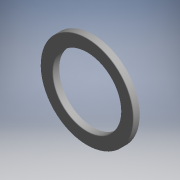
# Autodesk Inventor part: 51111 Housing raceway disc
Saved by Autodesk Inventor 2023 (Build 270158000, 158)
## iProperties
Part Number: 51111 Housing raceway disc
Material: 一般
Catalog Web Link: www.cadenas.de
Description: tb sdt hrd-
Vendor: NTN
Document SubType Name: Modeling
Designer: partserver
Manufacturer: NTN
Mass: 9.93491 g
Surface Area: 68.4869 cm^2
Volume: 9.93491 cm^3
Density: 1 g/cm^3
Appearance: PSOLRGB-192-192-192
Category: PARTsolutions
Company: NTN
PSOL_IDENT_0: {$CADENAS_DATA\23d-libs\ntn\ball_roller_bearings\thrust_b\tb_sdt_ir.prj},199 {VTYP=3D},{NB=51111 Hou
PSOL_IDENT_1: sing raceway disc},{LINA=51111 Housing raceway disc},{NN=tb sdt hrd},{DATE=21.12.2021 04:23:12},{GEO
PSOL_IDENT_2: MDATE=08.04.2020 13:27:59},{VERSION=},{LINEID=11140},{WBVAR=},{WBNUMERIC=}  {NB=51111 Housing racewa
PSOL_IDENT_3: y disc},{LINA=51111 Housing raceway disc},{KT=DUMMY},{IDNR=},{SD=55},{D=78},{T=16},{R=0.6},{ORDER=51
PSOL_IDENT_4: 111},{CA=35},{COA=93},{CAF=3 550},{COAF=9 500},{NG=2 800},{NO=4 000},{D1=78},{SD1=57},{MASS=0.23},{D
PSOL_IDENT_5: A1=69},{DA=64},{RAS=0,6},{X=10.50000},{BN=13.316964},{X1=11.50000},{O=208.81},{T1=5.33333},{T2=5.333
PSOL_IDENT_6: 33},{RB=4.48000}
NB: 51111 Housing raceway disc
NN: tb sdt hrd
NBSYN: $ORDER. Housing raceway disc
LINA: 51111 Housing raceway disc
CATALOG: NTN Corporation
SD: 55
D: 78
T: 16
R: 0.6
ORDER: 51111
CA: 35
COA: 93
CAF: 3 550
COAF: 9 500
NG: 2 800
NO: 4 000
D1: 78
SD1: 57
MASS: 0.23
DA1: 69
DA: 64
RAS: 0,6
SUPPLIER: NTN
ARTICLENO: 51111 Housing raceway disc
BOMINFO: 51111 Housing raceway disc
CREATOR: CADENAS GmbH
Title: 51111 Housing raceway disc
Author: Cadenas PARTsolutions
Autodesk Inventor part; units mm, degrees
sketch "Sketch_1" plane through (0, 0, 0) normal (0, 0, 1) x (1, 0, 0)
  line L0 (0, 5.3333) -> (0, 0)
  arc A0 (-39, 0.6) -> (-38.4, 0) centre (-38.4, 0.6) ccw
  line L1 (-38.4, 0) -> (-29.1, 0)
  arc A1 (-29.1, 0) -> (-28.5, 0.6) centre (-29.1, 0.6) ccw
  line L2 (-28.5, 0.6) -> (-28.5, 5.3333)
  line L3 (-28.5, 5.3333) -> (-29.6501, 5.3333)
  arc A2 (-36.8499, 5.3333) -> (-29.6501, 5.3333) centre (-33.25, 8) ccw
  line L4 (-36.8499, 5.3333) -> (-39, 5.3333)
  line L5 (-39, 5.3333) -> (-39, 0.6)
  constraints: 12 end point, 6 point on circle, 3 centre point
revolve "Revolution1" add sketch "Sketch_1" angle 360 about axis through (0, 5.3333, 0) along (0, 1, 0)
ref_plane "tb_sdt_hrd_XY" through (0, 0, 0) normal (0, 1, 0) x (1, 0, 0)
ref_plane "tb_sdt_hrd_YZ" through (0, 0, 0) normal (1, 0, 0) x (0, 0, -1)
ref_plane "tb_sdt_hrd_ZX" through (0, 0, 0) normal (0, 0, -1) x (0, 1, 0)
body "Solid1"
